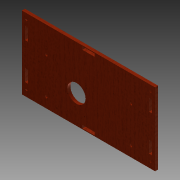
# Autodesk Inventor part: panStepperMountRB02
Saved by Autodesk Inventor 2013 (Build 170138000, 138)
## iProperties
Created: 2014-06-14
Part Number: panStepperMountRB02
Material: Wood (Oak)
Document SubType Name: Modeling
Designer: Byron
Density: 0.56 g/cm^3
Mass: 142.85 g
Surface Area: 867.195 cm^2
Volume: 255.089 cm^3
Author: Byron
Autodesk Inventor part; units mm, degrees
note: some values were not read from the file. Chosen so that the rebuilt part matches the saved one: pattern direction of "Rectangular Pattern1".
ref_plane "YZ Plane" through (0, 0, 0) normal (1, 0, 0) x (0, 1, 0)
ref_plane "XZ Plane" through (0, 0, 0) normal (0, 1, 0) x (-1, 0, 0)
ref_plane "XY Plane" through (0, 0, 0) normal (0, 0, 1) x (1, 0, 0)
sketch "Sketch1" plane through (0, 0, 0) normal (0, 0, 1) x (1, 0, 0)
  circle A0 centre (1.016, 0) radius 19.05
  line L0 (159.5437, -28.575) -> (159.5437, 29.0493) projected
  line L1 (145.8277, 86.9876) -> (-55.3403, 86.9876) projected
  line L2 (159.5437, 93.3376) -> (-107.1563, 93.3376)
  line L3 (-107.1563, 93.3376) -> (-107.1563, -59.0624)
  line L4 (-107.1563, -59.0624) -> (159.5437, -59.0624)
  line L5 (159.5437, -59.0624) -> (159.5437, 93.3376)
  point P0 (0, 0)
  dimension "d0" = 266.7
  dimension "d1" = 152.4
  dimension "d15" = 38.1
  constraints: 8 end point, 2 parallel, 1 centre point, 1 coincident, 1 horizontal, 1 perpendicular, 1 other
  measures "d0" distance of L3.end L4.end
  measures "d1" distance of L2.end L3.end
  measures "d15" diameter of A0
extrude "Extrusion1" add sketch "Sketch1" along normal blind 6.35
sketch "Sketch2" plane through (0, 0, 6.35) normal (0, 0, 1) x (1, 0, 0)
  line L0 (-107.1563, 93.3376) -> (159.5437, 93.3376) projected
  line L1 (-107.1563, -59.0624) -> (-107.1563, 93.3376) projected
  line L2 (-103.9813, 93.3376) -> (-103.9813, -59.0624) construction
  circle A0 centre (-103.9813, 80.6376) radius 1.8542
  dimension "d4" = 3.175
  dimension "d5" = 3.7084
  dimension "d6" = 12.7
  constraints: 2 end point, 1 centre point
  measures "d4" distance between parallel lines of L1 L2
  measures "d5" diameter of A0
  measures "d6" distance from line of L0 A0.centre
extrude "Extrusion2" cut sketch "Sketch2" against normal through all
pattern_linear "Rectangular Pattern1" count 2 spacing 127 along (0, -1, 0) count 2 spacing 260.35 along (1, 0, 0) of "Extrusion2"
sketch "Sketch3" plane through (0, 0, 0) normal (0, 0, -1) x (-1, 0, 0)
  circle A0 centre (62.484, 38.1) radius 2.5146 projected
  circle A1 centre (62.484, -38.1) radius 2.5146 projected
  circle A2 centre (-115.316, -38.1) radius 2.5146 projected
  circle A3 centre (-115.316, 38.1) radius 2.5146 projected
  point P0 (0, 0)
extrude "Extrusion3" cut sketch "Sketch3" against normal through all
sketch "Sketch4" plane through (0, 0, 0) normal (0, 0, -1) x (-1, 0, 0)
  line L0 (107.1563, 93.3376) -> (113.5063, 93.3376)
  line L1 (113.5063, 93.3376) -> (113.5063, -59.0624)
  line L2 (113.5063, -59.0624) -> (107.1563, -59.0624)
  line L3 (107.1563, -59.0624) -> (107.1563, 93.3376)
  line L4 (-159.5437, -59.0624) -> (-165.8937, -59.0624)
  line L5 (-165.8937, -59.0624) -> (-165.8937, 93.3376)
  line L6 (-165.8937, 93.3376) -> (-159.5437, 93.3376)
  line L7 (-159.5437, 93.3376) -> (-159.5437, -59.0624)
  point P0 (0, 0)
  dimension "d18" = 6.35
  dimension "d19" = 6.35
  constraints: 16 end point, 4 parallel, 2 horizontal, 2 perpendicular
  measures "d18" distance of L1.end L2.end
  measures "d19" distance of L5.end L6.end
extrude "Extrusion4" add sketch "Sketch4" against normal blind 6.35
sketch "Sketch5" plane through (0, 0, 0) normal (0, 0, -1) x (-1, 0, 0)
  line L0 (-159.5437, -59.0624) -> (-159.5437, 93.3376) projected
  line L1 (-159.5437, 93.3376) -> (-153.1937, 93.3376) projected
  line L2 (-153.1937, -59.0624) -> (-153.1937, 93.3376) projected
  line L3 (-159.5437, -59.0624) -> (-153.1937, -59.0624) projected
  line L4 (-159.5437, 68.2942) -> (-153.1937, 68.2942)
  line L5 (-153.1937, 68.2942) -> (-153.1937, 42.8942)
  line L6 (-153.1937, 42.8942) -> (-159.5437, 42.8942)
  line L7 (-159.5437, 42.8942) -> (-159.5437, 68.2942)
  line L8 (-159.5437, -7.9058) -> (-153.1937, -7.9058)
  line L9 (-153.1937, -7.9058) -> (-153.1937, -33.3058)
  line L10 (-153.1937, -33.3058) -> (-159.5437, -33.3058)
  line L11 (-159.5437, -33.3058) -> (-159.5437, -7.9058)
  line L12 (100.8063, 68.2942) -> (107.1563, 68.2942)
  line L13 (107.1563, 68.2942) -> (107.1563, 42.8942)
  line L14 (107.1563, 42.8942) -> (100.8063, 42.8942)
  line L15 (100.8063, 42.8942) -> (100.8063, 68.2942)
  line L16 (100.8063, -7.9058) -> (107.1563, -7.9058)
  line L17 (107.1563, -7.9058) -> (107.1563, -33.3058)
  line L18 (107.1563, -33.3058) -> (100.8063, -33.3058)
  line L19 (100.8063, -33.3058) -> (100.8063, -7.9058)
  point P0 (0, 0)
  dimension "d22" = 25.4
  dimension "d25" = 76.2
  dimension "d28" = 260.35
  constraints: 32 end point, 2 horizontal, 2 parallel, 1 collinear, 1 perpendicular, 1 vertical, 23 other
  measures "d22" distance of L4.end L5.end
  measures "d25" distance of L5.end L10.start
  measures "d28" distance of L5.end L14.start
extrude "Extrusion5" cut sketch "Sketch5" against normal through all contours L0 L8 L2 L10 | L0 L4 L2 L6 | L12 L13 L14 L15 | L16 L17 L18 L19
sketch "Sketch6" plane through (0, 0, 0) normal (0, 0, -1) x (-1, 0, 0)
  line L0 (-13.4937, 85.4001) -> (-13.4937, 91.7501) projected
  line L1 (-13.4937, 91.7501) -> (-38.8937, 91.7501) projected
  line L2 (-38.8937, 91.7501) -> (-38.8937, 85.4001) projected
  line L3 (-38.8937, 85.4001) -> (-13.4937, 85.4001) projected
  line L4 (-13.4937, -57.4749) -> (-13.4937, -51.1249) projected
  line L5 (-13.4937, -51.1249) -> (-38.8937, -51.1249) projected
  line L6 (-38.8937, -51.1249) -> (-38.8937, -57.4749) projected
  line L7 (-38.8937, -57.4749) -> (-13.4937, -57.4749) projected
  point P0 (0, 0)
extrude "Extrusion6" cut sketch "Sketch6" against normal through all
body "Solid1"
